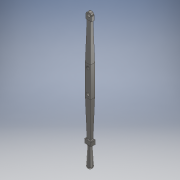
# Autodesk Inventor part: Eccentric Rod
Saved by Autodesk Inventor 2017 (Build 210142000, 142)
## iProperties
Created: 2018-11-18
Part Number: Eccentric Rod
Material: Stainless Steel
Document SubType Name: Modeling
Designer: Arman Grewal
Density: 8 g/cm^3
Appearance: Semi-Polished
Author: Arman Grewal
Autodesk Inventor part; units mm, degrees
ref_plane "YZ Plane" through (0, 0, 0) normal (1, 0, 0) x (0, 1, 0)
sketch "Sketch1" plane through (0, 0, 0) normal (0, 1, 0) x (-1, 0, 0)
  line L0 (0, 0) -> (0, -5) construction
  circle A0 centre (0, 0) radius 1.75 construction
  line L1 (0, 0) -> (-3.25, 0) construction
  line L2 (0, 0) -> (3.25, 0) construction
  line L3 (-3.25, 0) -> (-3.25, -5)
  line L4 (-3.25, -5) -> (3.25, -5)
  line L5 (3.25, -5) -> (3.25, 0)
  circle A1 centre (0, 0) radius 1.75
  arc A2 (3.25, 0) -> (-3.25, 0) centre (0, 0) ccw
  dimension "d1" = 5
  dimension "d2" = 3.5
  dimension "d3" = 3.25
  dimension "d4" = 3.25
  dimension "d5" = 3.5
  dimension "d6" = 5
  constraints: 12 end point, 3 centre point, 2 coincident, 2 horizontal, 2 perpendicular, 2 point on circle, 2 tangent, 2 vertical
  measures "d1" distance of L0.start L0.end
  measures "d2" diameter of A0
  measures "d3" distance of L1.start L1.end
  measures "d4" distance of L1.start L2.end
  measures "d5" diameter of A1
  measures "d6" distance between parallel lines of L2 L4
extrude "Extrusion1" add sketch "Sketch1" along normal blind 3
sketch "Sketch2" plane through (0, 0, 0) normal (1, 0, 0) x (0, 1, 0)
  line L0 (0, -5) -> (3, -5) construction
  line L1 (1.5, -5) -> (1.5, -48) construction
  line L2 (1.5, -5) -> (44.5, -5) construction
  line L3 (1.5, -48) -> (4, -48) construction
  line L4 (4, -48) -> (-1, -48) construction
  line L5 (4, -48) -> (-1, -48)
  line L6 (-1, -48) -> (-1, -83)
  line L7 (4, -48) -> (-1, -48)
  line L8 (-1, -48) -> (-1, -83)
  line L9 (-1, -83) -> (4, -83)
  line L10 (4, -83) -> (4, -48)
  point P0 (0, 0)
  dimension "d9" = 43
  dimension "d10" = 90
  dimension "d11" = 2.5
  dimension "d12" = 5
  dimension "d13" = 35
  constraints: 20 end point, 3 equal length, 3 horizontal, 3 perpendicular, 1 midpoint, 1 point on line, 1 vertical
  measures "d9" distance of L1.start L1.end
  measures "d10" angle of L1 L2
  measures "d11" distance of L1.end L3.end
  measures "d12" distance of L3.end L4.end
  measures "d13" distance of L4.end L6.end
extrude "Extrusion2" add sketch "Sketch2" along normal mid plane 6
sketch "Sketch3" plane through (3.25, 0, -5) normal (0, 0, -1) x (-1, 0, 0)
  line L0 (3.25, 0) -> (5.25, 0)
  line L1 (5.25, 0) -> (1.25, 0)
  line L2 (5.25, 0) -> (1.25, 0)
  line L3 (1.25, 0) -> (1.25, 3)
  line L4 (1.25, 3) -> (5.25, 3)
  line L5 (5.25, 3) -> (5.25, 0)
  dimension "d16" = 2
  dimension "d17" = 4
  dimension "d18" = 4
  dimension "d19" = 90
  dimension "d20" = 3
  constraints: 12 end point, 3 parallel, 1 horizontal, 1 perpendicular
  measures "d16" distance of L0.start L0.end
  measures "d17" distance of L0.end L1.end
  measures "d18" distance between parallel lines of L5 L3
  measures "d19" angle of L0 L5
  measures "d20" distance between parallel lines of L4 L2
loft "Loft1" add profiles "Sketch3" section 2 edges at (0, -1, -48) (3, 1.5, -48) (0, 4, -48) (-3, 1.5, -48)
sketch "Sketch4" plane through (-3, 4, -83) normal (0, 1, 0) x (1, 0, 0)
  circle A0 centre (3, -30.75) radius 1.75
  circle A1 centre (3, -4.25) radius 1.75
  line L0 (1, -78) -> (0, -35) construction
  line L1 (0, 0) -> (6, 0) construction
  line L2 (0, -35) -> (0, 0) construction
  line L3 (0, 0) -> (0, -35) construction
  line L4 (0, -17.5) -> (6, -17.5) construction
  line L5 (6, 0) -> (6, -35) construction
  line L6 (6, -35) -> (0, -35) construction
  point P0 (3, -83)
  point P1 (3, -35)
  dimension "d25" = 3.5
  dimension "d26" = 3.5
  dimension "d27" = 13.25
  dimension "d28" = 13.25
  constraints: 4 end point, 3 midpoint, 2 centre point, 2 vertical alignment, 1 vertical
  measures "d25" diameter of A0
  measures "d26" diameter of A1
  measures "d27" distance from line of L4 A0.centre
  measures "d28" distance from line of A1.centre L4
extrude "Extrusion3" cut sketch "Sketch4" against normal blind 6
fillet "Fillet1" radius 1 2 edges at (-2, 1.5, -5) (2, 1.5, -5)
thread "Thread1" size "M3.5x0.6" class "6H" standard "ANSI Metric M Profile" full length
ref_plane "Work Plane1" through (0, 0, -125) normal (0, 0, 1) x (1, 0, 0)
sketch "Sketch5" plane through (0, 0, -125) normal (0, 0, 1) x (1, 0, 0)
  line L0 (3, 4) -> (-3, 4) projected
  line L1 (0, 4) -> (4, 4)
  line L2 (4, 4) -> (-4, 4)
  line L3 (4, 4) -> (4, -1)
  line L4 (4, -1) -> (-4, -1)
  line L5 (-3, -1) -> (3, -1) projected
  line L6 (-4, -1) -> (-4, 4)
  point P0 (0, 0)
  dimension "d35" = 4
  dimension "d36" = 8
  dimension "d37" = 5
  constraints: 10 end point, 2 collinear, 1 midpoint, 1 perpendicular, 1 point on line, 1 vertical
  measures "d35" distance of L1.start L1.end
  measures "d36" distance of L1.end L2.end
  measures "d37" distance of L1.end L3.end
extrude "Extrusion4" add sketch "Sketch5" against normal blind 5
sketch "Sketch6" plane through (0, 0, -125) normal (0, 0, 1) x (1, 0, 0)
  line L0 (4, -1) -> (4, 4) projected
  line L1 (4, 1.5) -> (4, 3)
  line L2 (4, 1.5) -> (4, 0)
  line L3 (4, 4) -> (-4, 4) construction
  line L4 (0, 4) -> (0, 1.7266) construction
  line L5 (0, 3) -> (2, 3)
  line L6 (2, 3) -> (2, 0)
  line L7 (2, 0) -> (-2, 0)
  line L8 (-2, 0) -> (-2, 3)
  line L9 (-2, 3) -> (0, 3)
  point P0 (0, 0)
  dimension "d40" = 1.5
  dimension "d41" = 1.5
  dimension "d42" = 2
  dimension "d43" = 4
  dimension "d44" = 4
  dimension "d45" = 1
  dimension "d46" = 2.2734
  constraints: 16 end point, 4 perpendicular, 3 point on line, 2 midpoint, 1 collinear, 1 horizontal, 1 vertical
  measures "d40" distance of L1.start L1.end
  measures "d41" distance of L1.start L2.end
  measures "d42" distance of L5.start L5.end
  measures "d43" distance of L6.end L7.end
  measures "d44" distance between parallel lines of L3 L7
  measures "d45" distance between parallel lines of L3 L9
  measures "d46" distance from line of L4.end L3
loft "Loft2" add profiles "Sketch6" section 2 edges at (0, 4, -83) (3, 1.5, -83) (0, -1, -83) (-3, 1.5, -83)
fillet "Fillet2" radius 0.5 4 edges at (4, -1, -127.5) (4, 4, -127.5) (-4, -1, -127.5) (-4, 4, -127.5)
fillet "Fillet3" radius 0.8 2 edges at (-2, 1.5, -125) (2, 1.5, -125)
fillet "Fillet4" radius 0.5 6 edges at (-2.4059, 0, -125) (0, 0, -125) (2.4059, 0, -125) (-2.4096, 3, -125) (0, 3, -125) (2.4096, 3, -125)
fillet "Fillet5" radius 0.4 16 edges at (3.8536, 3.8536, -130) (4, 1.5, -130) (3.8536, -0.8536, -130) (0, -1, -130) (-3.8536, -0.8536, -130) (-4, 1.5, -130) (-3.8536, 3.8536, -130) (0, 4, -130) (-3.8536, 3.8536, -125) (-4, 1.5, -125) (-3.8536, -0.8536, -125) (0, -1, -125) (3.8536, -0.8536, -125) (4, 1.5, -125) (3.8536, 3.8536, -125) (0, 4, -125)
sketch "Sketch8" plane through (0, 0, -130) normal (0, 0, -1) x (-1, 0, 0)
  line L0 (-3.6, -0.5) -> (-3.6, 3.5) construction
  line L1 (-3.6, 1.5) -> (3.6, 1.5) construction
  line L2 (3.6, -0.5) -> (3.6, 3.5) construction
  circle A0 centre (0, 1.5) radius 2
  point P0 (0, 0)
  dimension "d58" = 4
  constraints: 3 midpoint, 2 end point, 1 centre point
  measures "d58" diameter of A0
ref_plane "Work Plane3" through (3.8828, 3.5, -154.8828) normal (0, 0, -1) x (-1, 0, 0)
sketch "Sketch9" plane through (3.8828, 3.5, -154.8828) normal (0, 0, -1) x (-1, 0, 0)
  circle A0 centre (3.8828, -2) radius 3.25
  line L0 (0.2828, -4) -> (0.2828, 0) projected
  point P0 (3.8828, -3.5)
  dimension "d60" = 6.5
  dimension "d61" = 1.5
  dimension "d62" = 3.6
  constraints: 1 centre point
  measures "d60" diameter of A0
  measures "d61" distance of A0.centre point (3.883, -3.5)
  measures "d62" distance from line of L0 A0.centre
loft "Loft3" add profiles "Sketch8", "Sketch9"
fillet "Fillet6" radius 3 1 edges at (3.25, 1.5, -154.8828)
fillet "Fillet7" radius 1 1 edges at (2, 1.5, -130)
body "Solid1"
